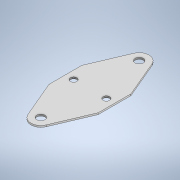
# Autodesk Inventor part: Platte2
Saved by Autodesk Inventor 2022 (Build 260153000, 153)
## iProperties
Created: 2022-04-02
Part Number: Platte2
Material: Generic
Document SubType Name: Modeling
Designer: benni
Density: 1 g/cm^3
Appearance: Default
Author: benni
Autodesk Inventor part; units mm, degrees
ref_plane "YZ Plane" through (0, 0, 0) normal (1, 0, 0) x (0, 1, 0)
ref_plane "XZ Plane" through (0, 0, 0) normal (0, 1, 0) x (-1, 0, 0)
ref_plane "XY Plane" through (0, 0, 0) normal (0, 0, 1) x (1, 0, 0)
sketch "Sketch1" plane through (0, 0, 0) normal (0, 1, 0) x (-1, 0, 0)
  line L0 (0, 0) -> (30, 0)
  line L1 (30, 0) -> (30, -20)
  line L2 (30, -20) -> (0, -20)
  line L3 (0, -20) -> (0, 0)
  line L4 (30, -10) -> (0, -10)
  line L5 (15, 0) -> (15, -20)
  circle A0 centre (25, -10) radius 2
  circle A1 centre (15, -40) radius 2.5
  circle A2 centre (5, -10) radius 2
  line L6 (30, 0) -> (0, 0)
  arc A3 (9.4763, -42.3428) -> (20.5237, -42.3428) centre (15, -40) ccw
  line L7 (30, -20) -> (20.5237, -42.3428)
  line L8 (0, -20) -> (9.4763, -42.3428)
  line L9 (30, 0) -> (0, 0)
  circle A4 centre (15, 20) radius 2.5
  arc A5 (20.5237, 22.3428) -> (9.4763, 22.3428) centre (15, 20) ccw
  line L10 (30, 0) -> (20.5237, 22.3428)
  line L11 (0, 0) -> (9.4763, 22.3428)
  dimension "d0" = 20
  dimension "d1" = 30
  dimension "d2" = 5
  dimension "d3" = 4
  dimension "d5" = 20
  dimension "d6" = 5
  dimension "d11" = 12
  constraints: 24 end point, 7 symmetric about line, 6 centre point, 5 coincident, 4 midpoint, 4 point on circle, 2 parallel, 1 horizontal, 1 perpendicular, 1 point on line, 1 tangent, 3 other
  measures "d0" distance of L0.end L1.end
  measures "d1" distance of L1.end L2.end
  measures "d2" distance from line of L1 point (25, -10)
  measures "d3" diameter of A0
  measures "d5" distance from line of L2 point (15, -40)
  measures "d6" diameter of A1
  measures "d11" diameter of A3
extrude "Extrusion2" add sketch "Sketch1" along normal blind 1 contours L11 A5 L10 L0 | L0 L5 L4 A2 L3 | L0 L1 L4 A0 L5 | L4 A2 L5 L2 L3 | L4 A0 L1 L2 L5 | L2 L7 A3 L8
body "Solid2"
